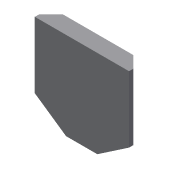
# Autodesk Inventor part: mount_bord
Saved by Autodesk Inventor 2014 SP1 (Build 180222100, 222)
## iProperties
Created: 2015-02-04
Part Number: mount_bord
Material: Generic
Document SubType Name: Modeling
Designer: Simen
Density: 1 g/cm^3
Appearance: Default
Author: Simen
Autodesk Inventor part; units mm, degrees
ref_plane "YZ Plane" through (0, 0, 0) normal (1, 0, 0) x (0, 1, 0)
ref_plane "XZ Plane" through (0, 0, 0) normal (0, 1, 0) x (-1, 0, 0)
ref_plane "XY Plane" through (0, 0, 0) normal (0, 0, 1) x (1, 0, 0)
sketch "Sketch1" plane through (0, 0, 0) normal (0, 1, 0) x (-1, 0, 0)
  line L0 (-23.8668, 27.2848) -> (413.1332, 27.2848)
  line L1 (413.1332, 27.2848) -> (413.1332, -379.7152)
  line L2 (413.1332, -379.7152) -> (-23.8668, -379.7152)
  line L3 (-23.8668, -379.7152) -> (-23.8668, 27.2848)
  line L4 (413.1332, -379.7152) -> (268.1332, -379.7152)
  line L5 (268.1332, -379.7152) -> (123.1332, -379.7152)
  line L6 (-23.8668, -379.7152) -> (-23.8668, -279.7152)
  line L7 (-23.8668, -279.7152) -> (123.1332, -379.7152)
  line L8 (268.1332, -379.7152) -> (413.1332, -279.7152)
  point P0 (0, 0)
  dimension "d0" = 437
  dimension "d1" = 407
  dimension "d2" = 145
  dimension "d3" = 145
  dimension "d4" = 100
  constraints: 18 end point, 4 point on line, 2 parallel, 1 horizontal, 1 perpendicular
  measures "d0" distance of L1.end L2.end
  measures "d1" distance of L0.end L1.end
  measures "d2" distance of L1.end L4.end
  measures "d3" distance of L4.end L5.end
  measures "d4" distance of L2.end L6.end
extrude "Extrusion1" add sketch "Sketch1" along normal blind 75 contours L0 L1 L8 L2 L7 L3
chamfer "Chamfer1" distance 55 angle 45 5 edges at (-49.6332, 75, -329.7152) (23.8668, 75, -126.2152) (-195.6332, 75, -379.7152) (-340.6332, 75, -329.7152) (-413.1332, 75, -126.2152)
body "Solid1"
